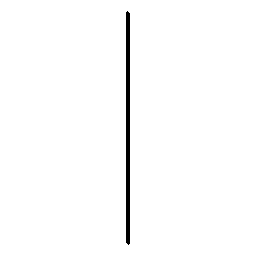
Reinforcement v14 (Autodesk Fusion 360 archive; units mm, degrees)
design "carbon fiber strip 1x5x500MM"
Autodesk Fusion 360 part; units mm, degrees
sketch "Sketch1" plane through (0, 0, 0) normal (0, 1, 0) x (1, 0, 0)
  line L0 (0, 0) -> (5, 0)
  line L1 (5, 0) -> (5, -1)
  line L2 (5, -1) -> (0, -1)
  line L3 (0, -1) -> (0, 0)
  dimension "d1" = 5
  dimension "d2" = 1
  constraint horizontal L0
  constraint vertical L1
  constraint horizontal L2
  constraint vertical L3
  constraint coincident L0.start L3.end
  measures "d1" distance of L0.start L0.end
  measures "d2" distance of L0.start L2.end
extrude "Extrude1" add sketch "Sketch1" along normal blind 500
fillet "Fillet1" radius 0.4 4 edges at (5, 250, 1) (0, 250, 1) (0, 250, 0) (5, 250, 0)
